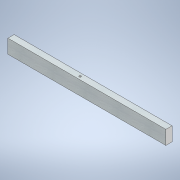
# Autodesk Inventor part: bodySidePlate
Saved by Autodesk Inventor 2021 (Build 250183000, 183)
## iProperties
Created: 2021-02-01
Part Number: bodySidePlate
Material: Generic
Document SubType Name: Modeling
Designer: garre
Density: 1 g/cm^3
Appearance: Default
Author: garre
Autodesk Inventor part; units mm, degrees
ref_plane "YZ Plane" through (0, 0, 0) normal (1, 0, 0) x (0, 1, 0)
ref_plane "XZ Plane" through (0, 0, 0) normal (0, 1, 0) x (-1, 0, 0)
ref_plane "XY Plane" through (0, 0, 0) normal (0, 0, 1) x (1, 0, 0)
sketch "Sketch1" plane through (0, 0, 0) normal (0, 0, 1) x (1, 0, 0)
  line L0 (0, 0) -> (647.7, 0)
  line L1 (647.7, 0) -> (647.7, 57.15)
  line L2 (647.7, 57.15) -> (0, 57.15)
  line L3 (0, 57.15) -> (0, 0)
  line L4 (647.7, 0) -> (647.7, 57.15)
  dimension "d0" = 647.7
  dimension "d1" = 57.15
  constraints: 10 end point, 2 parallel, 1 horizontal, 1 perpendicular
  measures "d0" distance of L1.end L2.end
  measures "d1" distance of L2.end L0.start
extrude "Extrusion1" add sketch "Sketch1" along normal blind 25.4
sketch "Sketch2" plane through (0, 0, 25.4) normal (0, 0, 1) x (1, 0, 0)
  line L0 (0, 0) -> (647.7, 0) projected
  line L1 (901.7, 0) -> (901.7, 25.4)
  line L2 (901.7, 25.4) -> (880.1227, 25.4)
  circle A0 centre (880.1227, 25.4) radius 17.399
  line L3 (880.1227, 25.4) -> (836.9681, 25.4)
  circle A1 centre (836.9681, 25.4) radius 17.399
  line L4 (836.9681, 25.4) -> (793.8135, 25.4)
  line L5 (793.8135, 25.4) -> (750.6589, 25.4)
  line L6 (750.6589, 25.4) -> (707.5043, 25.4)
  circle A2 centre (793.8135, 25.4) radius 17.399
  circle A3 centre (750.6589, 25.4) radius 17.399
  circle A4 centre (707.5043, 25.4) radius 17.399
  line L7 (901.7, 0) -> (901.7, 57.15) projected
  line L8 (901.7, 0) -> (901.7, 57.15)
  line L9 (707.5043, 25.4) -> (664.3497, 25.4)
  circle A5 centre (664.3497, 25.4) radius 9.525
  point P0 (787.6658, 25.1497)
  point P1 (813.0658, 25.1497)
  point P2 (838.4658, 25.1497)
  point P3 (863.8658, 25.1497)
  dimension "d7" = 25.4
  dimension "d8" = 21.5773
  dimension "d9" = 34.798
  dimension "d10" = 43.1546
  dimension "d13" = 19.05
  constraints: 16 end point, 6 centre point, 6 coincident, 5 collinear, 4 equal radius, 4 horizontal, 3 point on line
  measures "d7" distance of L1.start L1.end
  measures "d8" distance of L1.end L2.end
  measures "d9" diameter of A0
  measures "d10" distance of L3.start L3.end
  measures "d13" diameter of A5
extrude "Extrusion2" [suppressed]
sketch "Sketch3" plane through (0, 57.15, 0) normal (0, 1, 0) x (1, 0, 0)
  line L0 (0, 0) -> (0, -25.4) projected
  line L1 (0, 0) -> (283.972, 0)
  line L2 (283.972, 0) -> (283.972, -13.335)
  line L3 (283.972, -13.335) -> (0, -13.335)
  line L4 (0, -13.335) -> (0, 0)
  circle A0 centre (283.972, -13.335) radius 3.81
  dimension "d14" = 283.972
  dimension "d15" = 13.335
  dimension "d16" = 7.62
  constraints: 8 end point, 2 parallel, 1 centre point, 1 coincident, 1 horizontal, 1 perpendicular
  measures "d14" distance of L2.end L3.end
  measures "d15" distance of L1.end L2.end
  measures "d16" diameter of A0
extrude "Extrusion3" cut sketch "Sketch3" against normal blind 25.4 contours A0 L2 L3 | L3 L2 A0
equation "\"d0\" = bodyLengthUntilNut"
equation "\"d1\" = bodyHeight"
equation "\"d5\" = woodThickness"
equation "\"d7\" = motorHolesOffset"
equation "\"d8\" = motorHoleEndOffset"
equation "\"d9\" = motorHoleDiameter"
equation "\"d10\" = motorHoleSeparation"
equation "\"d13\" = wireHoleDiameter"
equation "\"bodyLengthUntilNut\" = 647.7"
equation "\"postNutAngle\" = 0"
equation "\"woodThickness\" = 25.4"
equation "\"slantLength\" = 127"
equation "\"extensionLength\" = 254"
equation "\"bodyHeight\" = 57.15"
equation "\"motorHolesOffset\" = 25.4"
equation "\"motorHoleEndOffset\" = 21.5773"
equation "\"motorHoleDiameter\" = 34.798"
equation "\"motorHoleSeparation\" = 43.1546"
equation "\"wireHoleDiameter\" = 19.05"
equation "\"temp\" = 0"
body "Solid1"
